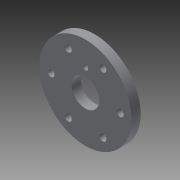
# Autodesk Inventor part: статор мотора
Saved by Autodesk Inventor 2013 (Build 170138000, 138)
## iProperties
Created: 2014-04-30
Part Number: статор мотора
Material: Типовые
Document SubType Name: Modeling
Designer: HP1
Density: 1 g/cm^3
Mass: 68.1726 g
Surface Area: 194.15 cm^2
Volume: 68.1726 cm^3
Author: HP1
Autodesk Inventor part; units mm, degrees
ref_plane "YZ Plane" through (0, 0, 0) normal (1, 0, 0) x (0, 1, 0)
ref_plane "XZ Plane" through (0, 0, 0) normal (0, 1, 0) x (-1, 0, 0)
ref_plane "XY Plane" through (0, 0, 0) normal (0, 0, 1) x (1, 0, 0)
sketch "Эскиз1" plane through (0, 0, 0) normal (0, 1, 0) x (-1, 0, 0)
  circle A0 centre (0, 0) radius 15
  circle A1 centre (0, 0) radius 50
  circle A2 centre (37.5, 0) radius 4
  circle A3 centre (18.75, 32.476) radius 4
  circle A4 centre (-18.75, 32.476) radius 4
  circle A5 centre (-37.5, 0) radius 4
  circle A6 centre (-18.75, -32.476) radius 4
  circle A7 centre (18.75, -32.476) radius 4
  circle A8 centre (0, 24) radius 3
  circle A9 centre (0, 0) radius 25 construction
  line L0 (41.5, -3.7528) -> (35, -7.5056) construction
  line L1 (35, -7.5056) -> (28.5, -3.7528) construction
  line L2 (28.5, -3.7528) -> (28.5, 3.7528) construction
  line L3 (28.5, 3.7528) -> (35, 7.5056) construction
  line L4 (35, 7.5056) -> (41.5, 3.7528) construction
  line L5 (41.5, 3.7528) -> (41.5, -3.7528) construction
  point P0 (35.3864, 0)
  point P1 (35, 0)
  dimension "d0" = 30
  dimension "d1" = 100
  dimension "d2" = 8
  dimension "d6" = 360
  dimension "d8" = 6
  dimension "d9" = 24
  dimension "d12" = 37.5
  dimension "d13" = 50
  dimension "d15" = 13
  constraints: 12 end point, 10 centre point, 1 concentric, 26 other
  measures "d0" diameter of A0
  measures "d1" diameter of A1
  measures "d2" diameter of A2
  measures "d8" diameter of A8
  measures "d9" distance of point (0, 0) A8.centre
  measures "d12" distance of A2.centre A0.centre
  measures "d13" diameter of A9
  measures "d15" distance between parallel lines of L2 L5
extrude "Выдавливание1" add sketch "Эскиз1" along normal blind 10
